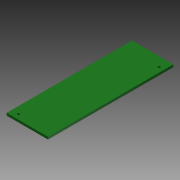
# Autodesk Inventor part: Yagi_Board
Saved by Autodesk Inventor 2014 (Build 180170000, 170)
## iProperties
Created: 2015-01-07
Part Number: Yagi_Board
Material: Generic
Document SubType Name: Modeling
Designer: Owner
Density: 1 g/cm^3
Appearance: Smooth - Dark Forest Green
Author: Owner
Autodesk Inventor part; units mm, degrees
ref_plane "YZ Plane" through (0, 0, 0) normal (1, 0, 0) x (0, 1, 0)
ref_plane "XZ Plane" through (0, 0, 0) normal (0, 1, 0) x (-1, 0, 0)
ref_plane "XY Plane" through (0, 0, 0) normal (0, 0, 1) x (1, 0, 0)
sketch "Sketch1" plane through (0, 0, 0) normal (0, 1, 0) x (-1, 0, 0)
  line L0 (16.4975, 25.7055) -> (44.1835, 25.7055)
  line L1 (44.1835, 25.7055) -> (44.1835, -58.1145)
  line L2 (44.1835, -58.1145) -> (16.4975, -58.1145)
  line L3 (16.4975, -58.1145) -> (16.4975, 25.7055)
  point P0 (0, 0)
  dimension "d0" = 27.686
  dimension "d1" = 83.82
  constraints: 8 end point, 2 parallel, 1 horizontal, 1 perpendicular
  measures "d0" distance of L0.start L0.end
  measures "d1" distance of L0.end L1.end
extrude "Extrusion1" add sketch "Sketch1" along normal blind 1.6
sketch "Sketch2" plane through (0, 1.6, 0) normal (0, 1, 0) x (1, 0, 0)
  line L0 (-44.1835, -25.7055) -> (-16.4975, -25.7055) projected
  line L1 (-16.4975, -25.7055) -> (-16.4975, 58.1145) projected
  line L2 (-16.4975, 58.1145) -> (-44.1835, 58.1145) projected
  line L3 (-44.1835, 58.1145) -> (-44.1835, -25.7055) projected
  circle A0 centre (-19.6725, 51.7645) radius 0.7937
  circle A1 centre (-39.421, -22.5305) radius 0.7938
  point P0 (0, 0)
  dimension "d4" = 1.5875
  dimension "d5" = 1.5875
  dimension "d6" = 3.175
  dimension "d7" = 4.7625
  dimension "d8" = 6.35
  dimension "d9" = 3.175
  constraints: 2 centre point
  measures "d4" diameter of A0
  measures "d5" diameter of A1
  measures "d6" distance from line of L0 A1.centre
  measures "d7" distance from line of L3 A1.centre
  measures "d8" distance from line of L2 A0.centre
  measures "d9" distance from line of L1 A0.centre
extrude "Extrusion2" cut sketch "Sketch2" against normal up to next contours A0 | A1
body "Solid1"
